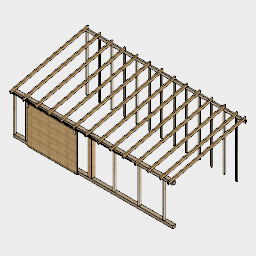
Doro4 Workshop v17 (Autodesk Fusion 360 design; units mm, degrees)
Autodesk Fusion 360 part; units mm, degrees
note: some values were not read from the file. Chosen so that the rebuilt part matches the saved one: which face or edge a step refers to. Set by a fixed rule: which sketch regions a step uses.
sketch "Sketch6" plane through (0, 0, 0) normal (0, 0, 1) x (1, 0, 0)
  line L0 (0, 0) -> (8000, 0)
  line L1 (8000, 0) -> (8000, 120)
  line L2 (8000, 120) -> (0, 120)
  line L3 (0, 120) -> (0, 0)
  dimension "d47" = 8000
  dimension "d51" = 120
  measures "d47" distance of L0.start L0.end
  measures "d51" distance of L0.start L2.end
extrude "Extrude1" add sketch "Sketch6" along normal blind 2200 makes body 1 in component "brick wall"
sketch "Sketch7" plane through (0, 0, 0) normal (1, 0, 0) x (0, 1, 0)
  line L0 (-3775, 0) -> (-3625, 0)
  line L1 (-3625, 0) -> (-3625, -50)
  line L2 (-3625, -50) -> (-3775, -50)
  line L3 (-3775, -50) -> (-3775, 0)
  line L4 (-3700, 0) -> (-3700, -50) construction
  dimension "d52" = 150
  dimension "d53" = 50
  dimension "d56" = 3700
  measures "d52" distance of L0.start L0.end
  measures "d53" distance of L0.start L2.end
  measures "d56" distance of origin L4
extrude "Extrude1'" add sketch "Sketch7" along normal blind 8000 separate body makes body 2 in component "concrete sleepers"
sketch "Sketch8" plane through (0, 0, 0) normal (0, 0, 1) x (1, 0, 0)
  line L0 (-1000, 1000) -> (10000, 1000)
  line L1 (10000, 1000) -> (10000, -7000)
  line L2 (10000, -7000) -> (-1000, -7000)
  line L3 (-1000, -7000) -> (-1000, 1000)
extrude "Extrude1''" add sketch "Sketch8" against normal blind 500 separate body makes body 3 in component "sand"
combine "Combine1" operation cut target body 3 tool bodies 2 keep tools in component "sand"
sketch "Sketch9" plane through (0, 0, 0) normal (1, 0, 0) x (0, 1, 0)
  line L0 (0, 0) -> (-60, 0)
  line L1 (-60, 0) -> (-60, 3000)
  line L2 (-60, 3000) -> (0, 3000)
  line L3 (0, 3000) -> (0, 0)
  line L4 (-3700, 0) -> (-3600, 0)
  line L5 (-3600, 0) -> (-3600, 2150)
  line L6 (-3600, 2150) -> (-3700, 2150)
  line L7 (-3700, 2150) -> (-3700, 0)
  line L8 (-3600, 2150) -> (0, 3000)
  line L9 (-3600, 2150) -> (-3745.9859, 2115.5311)
  line L10 (0, 3000) -> (146.9725, 3034.7018)
  line L11 (120, 0) -> (120, 2200)
  line L12 (-3745.9859, 2115.5311) -> (-3718.4108, 1998.7423)
  line L13 (-3718.4108, 1998.7423) -> (146.9725, 2911.4023)
  line L14 (146.9725, 3034.7018) -> (146.9725, 2911.4023)
  line L15 (146.9725, 3034.7018) -> (141.2276, 3059.0328)
  line L16 (141.2276, 3059.0328) -> (-3849.0547, 2116.8828)
  line L17 (-3849.0547, 2116.8828) -> (-3843.3099, 2092.5518)
  line L18 (-3843.3099, 2092.5518) -> (146.9725, 3034.7018)
  line L19 (-3775, 0) -> (-3625, 0)
  line L20 (0, 2876.7005) -> (-60, 2876.7005)
  line L21 (-60, 2876.7005) -> (-60, 2756.7005)
  line L22 (-60, 2756.7005) -> (0, 2756.7005)
  line L23 (0, 2756.7005) -> (0, 2876.7005)
  line L24 (-3760, 2112.2222) -> (-3600, 2112.2222)
  line L25 (-3600, 2112.2222) -> (-3600, 1952.2222)
  line L26 (-3600, 1952.2222) -> (-3760, 1952.2222)
  line L27 (-3760, 1952.2222) -> (-3760, 2112.2222)
  line L28 (-3575, 2032.6032) -> (-3575, 1952.6032)
  line L29 (-3575, 1952.6032) -> (-3600, 1952.6032)
  point P0 (-3775, 0)
  dimension "d59" = 3000
  dimension "d60" = 60
  dimension "d61" = 2150
  dimension "d62" = 100
  dimension "d63" = 3700
  dimension "d65" = 150
  dimension "d66" = 4000
  dimension "d69" = 13.144
  dimension "d70" = 120
  dimension "d71" = 25
  dimension "d73" = 4100
  dimension "d105" = 60
  dimension "d106" = 120
  dimension "d123" = 160
  dimension "d124" = 160
  dimension "d125" = 80
  dimension "d126" = 25
  measures "d59" distance of L0.start L2.end
  measures "d60" distance of L0.start L0.end
  measures "d61" distance of L4.start L6.end
  measures "d62" distance of L4.start L4.end
  measures "d63" distance of L3 L7
  measures "d65" distance of L5.end L9.end
  measures "d66" distance of L9.end L10.end
  measures "d70" distance of L9.end L12.end
  measures "d71" distance of L10.end L15.end
  measures "d73" distance of L15.end L16.end
  measures "d105" distance of L20.start L20.end
  measures "d106" distance of L20.start L22.end
  measures "d123" distance of L24.start L24.end
  measures "d124" distance of L24.start L26.end
  measures "d125" distance of L28.start L28.end
  measures "d126" distance of L28.end L29.end
extrude "Extrude1'''" add sketch "Sketch9" along normal blind 60 separate body contours L0 L1 L3 L22 | L5 L7 L13 L24 L25 | L5 L7 L13 L25 L26 | L6 L7 L9 L18 | L5 L7 L9 L18 L24 | L4 L5 L7 L19 L26 makes body 4 at (0, -3666.6667, 716.6667) makes body 5 at (40, -60, 918.9002) in component "posts"
copy_body "Body->Comp1" bodies 5 removing the originals makes body 6 in component "KVH 60x60 back"
copy_body "Body->Comp2" bodies 4 removing the originals makes body 7 in component "KVH 100x100 front"
extrude "Extrude1''''" add sketch "Sketch9" along normal blind 60 separate body contours L1 L3 L8 L18 L20 | L3 L10 L13 L14 L18 | L1 L5 L8 L13 L18 L21 L25 | L5 L7 L13 L24 L25 | L5 L7 L9 L18 L24 | L7 L12 L13 L24 | L7 L9 L12 L18 L24 makes body 8 in component "rafter"
extrude "Extrude1'''''" add sketch "Sketch9" along normal blind 8000 separate body contours L1 L2 L8 L18 | L1 L2 L6 L7 L8 L9 L10 L15 L16 L17 L18 | L6 L7 L9 L18 makes body 9 in component "roof deck OSB 25mm"
extrude "Extrude1''''''" add sketch "Sketch9" along normal blind 8000 separate body contours L5 L7 L13 L24 L25 | L5 L7 L13 L25 L26 | L7 L12 L13 L24 | L7 L12 L13 L24 L26 L27 makes body 10 in component "top plate BSH 130x180"
extrude "Extrude1'''''''" add sketch "Sketch9" along normal blind 60 separate body contours L1 L5 L8 L13 L18 L21 L25 makes body 11 in component "knagge OSB 25mm"
extrude "Extrude1''''''''" add sketch "Sketch9" along normal blind 8000 separate body contours L5 L13 L25 L28 L29 makes body 12 in component "sleeper KVH 40x60"
extrude "Extrude1'''''''''" add sketch "Sketch9" along normal blind 8000 separate body contours L1 L3 L13 L21 L22 L23 | L1 L13 L20 L21 makes body 13 in component "top plate KVH 40x60"
sketch "Sketch10" plane through (0, 120, 0) normal (0, 1, 0) x (-1, 0, 0)
  line L0 (-8000, 2100) -> (0, 2100)
  line L1 (0, 2100) -> (0, 3050)
  line L2 (0, 3050) -> (-8000, 3050)
  line L3 (-8000, 3050) -> (-8000, 2100)
  dimension "d107" = 8000
  dimension "d108" = 950
  measures "d107" distance of L0.start L0.end
  measures "d108" distance of L0.start L2.end
extrude "Extrude1''''''''''" add sketch "Sketch10" along normal blind 12 separate body makes body 14 in component "OSB 12mm"
pattern_linear "R-Pattern1" [suppressed] in component "rafters"
sketch "Sketch11" plane through (0, 0, 0) normal (0, 0, -1) x (1, 0, 0)
  line L0 (3750, 3700) -> (3750, 3600)
  line L1 (3750, 3600) -> (3810, 3600)
  line L2 (3810, 3600) -> (3810, 3700)
  line L3 (3810, 3700) -> (3750, 3700)
  line L4 (3750, 3700) -> (3930, 3700)
  line L5 (3930, 3700) -> (3930, 3520)
  line L6 (3930, 3520) -> (3750, 3520)
  line L7 (3750, 3520) -> (3750, 3700)
  dimension "d115" = 180
  dimension "d116" = 180
  measures "d115" distance of L0.start L4.end
  measures "d116" distance of L0.start L6.end
extrude "Extrude1'''''''''''" add sketch "Sketch11" against normal blind 1984.124 separate body makes body 15 in component "post BSH 180x180"
combine "Combine1'" operation cut target body 15 tool bodies 12 10 keep tools in component "post BSH 180x180"
pattern_linear "R-Pattern1'" [suppressed] in component "posts west"
sketch "Sketch12" plane through (0, 0, 0) normal (0, 0, 1) x (1, 0, 0)
move_face "OffsetFaces1" offset -272.7778 1 faces at (20, -3633.3333, 2150) on bodies 7 in component "KVH 100x100 front"
sketch "Sketch13" plane through (0, 0, 0) normal (-1, 0, 0) x (0, -1, 0)
  line L0 (3760, 1952.2222) -> (3760, 2112.2222)
  line L1 (3600, 1952.2222) -> (3760, 1952.2222)
  line L2 (3760, 1952.2222) -> (3790, 1952.2222)
  line L3 (3790, 1952.2222) -> (3790, 1982.2222)
  line L4 (3760, 1982.2222) -> (3760, 1952.2222)
  line L5 (3786, 1956.2222) -> (3764, 1956.2222)
  line L6 (3764, 1956.2222) -> (3764, 1982.2222)
  line L7 (3786, 1982.2222) -> (3786, 1956.2222)
  line L8 (3764, 1982.2222) -> (3760, 1982.2222)
  line L9 (3786.0001, 1982.5) -> (3790.0001, 1982.5)
  line L10 (3790.0001, 1982.5) -> (3790.0001, 2022.5)
  line L11 (3790.0001, 2022.5) -> (3786.0001, 2022.5)
  line L12 (3786.0001, 2022.5) -> (3786.0001, 1982.5)
  line L13 (3795, 1975) -> (3781.0001, 1975)
  line L14 (3781.0001, 1975) -> (3781.0001, 2030.0001)
  line L15 (3781.0001, 2030.0001) -> (3795, 2030.0001)
  line L16 (3795, 2030.0001) -> (3795, 1975)
  line L17 (3795, 1975) -> (3781.0001, 2030.0001) construction
  line L18 (3781.0001, 1975) -> (3795, 2030.0001) construction
  line L19 (3795, 1975) -> (3794.0001, 1975)
  line L20 (3794.0001, 1975) -> (3790.0001, 1982.5)
  line L21 (3781.0001, 1975) -> (3782.0001, 1975)
  line L22 (3786.0001, 1982.5) -> (3782.0001, 1975)
  line L23 (3781.0001, 2002.5) -> (3795, 2002.5)
  line L24 (3786, 1982.2222) -> (3790, 1982.2222)
  line L25 (3795, 1998.5) -> (3781.0001, 1998.5)
  line L26 (3781.0001, 1998.5) -> (3781.0001, 2006.5)
  line L27 (3781.0001, 2006.5) -> (3795, 2006.5)
  line L28 (3795, 2006.5) -> (3795, 1998.5)
  line L29 (3795, 1998.5) -> (3781.0001, 2006.5) construction
  line L30 (3781.0001, 1998.5) -> (3795, 2006.5) construction
  line L31 (3760, 1940) -> (3785, 1940)
  line L32 (3785, 1940) -> (3785, 40)
  line L33 (3785, 40) -> (3760, 40)
  line L34 (3760, 40) -> (3760, 1940)
  line L35 (3760, 1940) -> (3720, 1940)
  line L36 (3720, 1940) -> (3720, 1880)
  line L37 (3720, 1880) -> (3760, 1880)
  line L38 (3760, 1880) -> (3760, 1940)
  line L39 (3760, 40) -> (3720, 40)
  line L40 (3720, 40) -> (3720, 100)
  line L41 (3720, 100) -> (3760, 100)
  line L42 (3760, 100) -> (3760, 40)
  line L43 (3777.0001, 1989.4383) -> (3777.0001, 2032)
  line L44 (3799.0001, 2032) -> (3799.0001, 1732)
  arc A0 (3799.0001, 2032) -> (3777.0001, 2032) centre (3788.0001, 2032) ccw
  line L45 (3775.5001, 1989.4383) -> (3775.5001, 2032)
  arc A1 (3800.5001, 2032) -> (3775.5001, 2032) centre (3788.0001, 2032) ccw
  line L46 (3800.5001, 2032) -> (3800.5001, 1732)
  line L47 (3775.5001, 1989.4383) -> (3777.0001, 1989.4383)
  line L48 (3799.0001, 1732) -> (3800.5001, 1732)
  point P0 (3788.0001, 2002.5)
  point P1 (3788.0001, 2002.5)
  dimension "d128" = 30
  dimension "d129" = 30
  dimension "d132" = 40
  dimension "d134" = 8
  dimension "d135" = 25
  dimension "d136" = 1900
  dimension "d137" = 60
  dimension "d138" = 40
  dimension "d139" = 40
  dimension "d140" = 60
  dimension "d141" = 300
  dimension "d142" = 1.5
  measures "d128" distance of L0.start L2.end
  measures "d129" distance of L0.start L4.start
  measures "d132" distance of L9.start L11.end
  measures "d134" distance of L25.end L26.end
  measures "d135" distance of L31.start L31.end
  measures "d136" distance of L31.start L33.end
  measures "d137" distance of L31.start L37.end
  measures "d138" distance of L31.start L35.end
  measures "d139" distance of L33.end L39.end
  measures "d140" distance of L33.end L41.end
  measures "d141" distance of L44.start L44.end
extrude "Extrude1''''''''''''" add sketch "Sketch13" against normal blind 6000 separate body contours L0 L2 L3 L4 L5 L6 L7 L8 L13 | L3 L7 L13 L24 makes body 16 in component "Component''"
extrude "Extrude1'''''''''''''" add sketch "Sketch13" against normal blind 60 separate body contours L43 L44 A0 L45 A1 L46 L47 L48 makes body 17 in component "Component'''"
revolve "Revolve1" add sketch "Sketch13" angle 360 about axis through (0, -3781.0001, 2002.5) along (0, -1, 0) separate body contours L10 L13 L16 L19 L20 L25 | L9 L10 L12 L25 | L12 L13 L14 L21 L22 L25 makes body 18 in component "Component''''"
extrude "Extrude1''''''''''''''" add sketch "Sketch13" against normal blind 2500 separate body contours L31 L32 L33 L34 L38 L42 makes body 19 in component "Component'''''"
extrude "Extrude1'''''''''''''''" add sketch "Sketch13" against normal blind 2500 separate body contours L34 L35 L36 L37 L38 | L34 L39 L40 L41 L42 makes body 20 at (833.3333, -3760, 1900) makes body 21 at (833.3333, -3760, 60) in component "Component''''''"
move_face "OffsetFaces1'" offset -30 3 faces at (2666.6667, -3666.6667, 2112.2222) (2666.6667, -3730.1365, 2112.2222) (5333.3333, -3755.0682, 2112.2222) on bodies 10 in component "top plate BSH 130x180"
sketch "Sketch14" plane through (7560, 0, 0) normal (1, 0, 0) x (0, 1, 0)
  line L0 (-3700, 0) -> (-3700, 2550)
  line L1 (0, 0) -> (0, 3450)
  line L2 (0, 3450) -> (-3700, 2550)
  line L3 (0, 0) -> (-3700, 0)
  dimension "d153" = 2550
  dimension "d154" = 3450
  measures "d153" distance of L0.start L0.end
  measures "d154" distance of L1.start L1.end
extrude "Extrude1''''''''''''''''" add sketch "Sketch9" along normal blind 8000 separate body contours L5 L7 L13 L24 L25 | L5 L7 L13 L25 L26 | L7 L12 L13 L24 | L7 L12 L13 L24 L26 L27 makes body 22 in component "top plate BSH 130x180 (1)"
move_face "OffsetFaces1''" offset -30 3 faces at (2666.6667, -3666.6667, 2112.2222) (2666.6667, -3730.1365, 2112.2222) (5333.3333, -3755.0682, 2112.2222) on bodies 22 in component "top plate BSH 130x180 (1)"
move_face "OffsetFaces2" offset -130 1 faces at (20, -3666.6667, 0) on bodies 7 in component "KVH 100x100 front"
move_face "OffsetFaces1'''" offset -130 1 faces at (3810, -3640, 0) on bodies 15 in component "post BSH 180x180"
move_face "OffsetFaces1''''" offset -145 1 faces at (20, 146.9725, 2993.602) on bodies 8 in component "rafter"
move_face "OffsetFaces2'" offset 145 2 faces at (20, -3736.2734, 2074.3956) (20, -3745.7255, 2114.4281) on bodies 8 in component "rafter"
extrude "Extrude1'''''''''''''''''" [suppressed] in component "Frame Element"
extrude "Extrude1''''''''''''''''''" [suppressed]
extrude "Extrude2" [suppressed]
sketch "Sketch2" plane through (8100, 0, 0) normal (1, 0, 0) x (0, 1, 0)
  line L0 (-2950, 0) -> (-2950, 2000)
  line L1 (-3450, 0) -> (-3450, 2000)
  line L2 (-2950, 0) -> (-3450, 0)
  line L3 (-2950, 2000) -> (-3450, 2000)
  line L4 (-3450, 0) -> (-3400, 0)
  line L5 (-3400, 0) -> (-3400, 2550)
  line L6 (-3400, 2550) -> (-3450, 2550)
  line L7 (-3450, 2550) -> (-3450, 0)
  line L8 (-100, 0) -> (0, 0)
  line L9 (-100, 0) -> (-100, 2000)
  line L10 (0, 2000) -> (-100, 2000)
  line L11 (0, 0) -> (0, 2000)
  line L12 (-100, 2000) -> (-3450, 2550)
  line L13 (-3450, 2550) -> (-3420.8382, 2727.622)
  line L14 (-100, 2000) -> (-70.8382, 2177.622)
  line L15 (-70.8382, 2177.622) -> (-3420.8382, 2727.622)
  line L16 (-70.8382, 2177.622) -> (-41.2345, 2172.7617)
  line L17 (-41.2345, 2172.7617) -> (0, 2000)
  line L18 (-3420.8382, 2727.622) -> (-3618.196, 2760.0241)
  line L19 (-3450, 2550) -> (-3548.6789, 2566.201)
  line L20 (-3618.196, 2760.0241) -> (-3627.9166, 2700.8167)
  line L21 (-3627.9166, 2700.8167) -> (-3548.6789, 2566.201)
  line L22 (-3450, 0) -> (-3500, 0)
  line L23 (-3500, 0) -> (-3500, 2550)
  line L24 (-3500, 2550) -> (-3450, 2550)
  line L25 (-3450, 2550) -> (-3450, 0)
  dimension "d16" = 2550
  dimension "d17" = 50
  dimension "d18" = 180
  dimension "d19" = 180
  dimension "d20" = 30
  dimension "d21" = 200
  dimension "d22" = 100
  dimension "d23" = 60
  dimension "d26" = 50
  dimension "d46" = 2550
  measures "d16" distance of L1.start L6.end
  measures "d17" distance of L1.start L4.end
  measures "d18" distance of L6.end L13.end
  measures "d19" distance of L9.end L14.end
  measures "d20" distance of L14.end L16.end
  measures "d21" distance of L13.end L18.end
  measures "d22" distance of L6.end L19.end
  measures "d23" distance of L18.end L20.end
  measures "d26" distance of L1.start L22.end
  measures "d46" distance of L22.end L23.end
extrude "Extrude3" [suppressed]
copy_body "CutPasteBodies1" [suppressed] in component "Frame Element"
extrude "Extrude4" [suppressed]
copy_body "CutPasteBodies2" [suppressed] in component "Frame Element"
sketch "Sketch3" plane through (0, 802.823, 1792.9713) normal (0, 0.408665, 0.912685) x (-1, 0, 0)
  line L0 (-8100, 4779.0884) -> (-8040, 4779.0884)
  line L1 (-8100, 4779.0884) -> (-8100, 4679.0884)
  line L2 (-8040, 4679.0884) -> (-8040, 4779.0884)
  line L3 (-8100, 4579.0884) -> (-8100, 4679.0884)
  line L4 (-8040, 4579.0884) -> (-8040, 4679.0884)
  line L5 (-8100, 4533.4541) -> (-8100, 4579.0884)
  line L6 (-8040, 4533.4541) -> (-8040, 4579.0884)
  line L7 (-8100, 4524.3049) -> (-8100, 4533.4541)
  line L8 (-8040, 4524.3049) -> (-8040, 4533.4541)
  line L9 (-8100, 908.5979) -> (-8100, 4524.3049)
  line L10 (-8040, 908.5979) -> (-8040, 4524.3049)
  line L11 (-8100, 817.3295) -> (-8100, 908.5979)
  line L12 (-8040, 817.3295) -> (-8040, 908.5979)
  line L13 (-8100, 817.3295) -> (-8040, 817.3295)
  line L14 (-8100, 4779.0884) -> (400, 4779.0884)
  line L15 (400, 4779.0884) -> (400, 1279.0884)
  line L16 (400, 1279.0884) -> (-8100, 1279.0884)
  line L17 (-8100, 1279.0884) -> (-8100, 4779.0884)
  dimension "d27" = 3500
  dimension "d28" = 8500
  measures "d27" distance of L0.start L16.end
  measures "d28" distance of L0.start L14.end
extrude "Extrude1'''''''''''''''''''" [suppressed] in component "Component"
pattern_linear "R-Pattern1''" [suppressed]
sketch "Sketch4" plane through (-333.3333, 0, 0) normal (-1, 0, 0) x (0, -1, 0)
  line L0 (0, 0) -> (625, 0)
  line L1 (625, 0) -> (625, 2050)
  line L2 (625, 2050) -> (0, 2050)
  line L3 (0, 2050) -> (0, 0)
  dimension "d35" = 625
  dimension "d36" = 2050
  measures "d35" distance of L0.start L0.end
  measures "d36" distance of L0.start L2.end
extrude "Extrude1''''''''''''''''''''" [suppressed] in component "Component'"
sketch "Sketch5" plane through (0, -3500, 0) normal (0, -1, 0) x (1, 0, 0)
  line L0 (8100, 0) -> (5600, 0)
  line L1 (5600, 0) -> (5600, 1250)
  line L2 (5600, 1250) -> (8100, 1250)
  line L3 (8100, 1250) -> (8100, 0)
  dimension "d39" = 2500
  dimension "d40" = 1250
  measures "d39" distance of L0.start L0.end
  measures "d40" distance of L0.start L2.end
extrude "Extrude1'''''''''''''''''''''" [suppressed] in component "OSB 15mm 2500x1250"
extrude "Extrude1''''''''''''''''''''''" [suppressed] in component "OSB 15mm 2500x1250 (1)"
move_face "OffsetFaces1'''''" [suppressed] in component "OSB 15mm 2500x1250 (1)"
extrude "Extrude1'''''''''''''''''''''''" [suppressed] in component "OSB 15mm 2500x1250 (2)"
move_face "OffsetFaces1''''''" [suppressed] in component "OSB 15mm 2500x1250 (2)"
component "brick wall" placed x (1, 0, 0) y (0, 1, 0) z (0, 0, 1) at (0, 0, 0)
component "concrete sleepers" placed x (1, 0, 0) y (0, 1, 0) z (0, 0, 1) at (0, 0, 0)
component "sand" placed x (1, 0, 0) y (0, 1, 0) z (0, 0, 1) at (0, 0, 0)
component "posts" placed x (1, 0, 0) y (0, 1, 0) z (0, 0, 1) at (0, 0, 0)
component "rafter" placed x (1, 0, 0) y (0, 1, 0) z (0, 0, 1) at (0, 0, 0)
component "roof deck OSB 25mm" placed x (1, 0, 0) y (0, 1, 0) z (0, 0, 1) at (0, 0, 0)
component "top plate BSH 130x180" placed x (1, 0, 0) y (0, 1, 0) z (0, 0, 1) at (0, 60, -75)
component "sleeper KVH 40x60" placed x (1, 0, 0) y (0, 1, 0) z (0, 0, 1) at (0, 0, 0)
component "top plate KVH 40x60" placed x (1, 0, 0) y (0, 1, 0) z (0, 0, 1) at (0, 0, 0)
component "OSB 12mm" placed x (1, 0, 0) y (0, 1, 0) z (0, 0, 1) at (0, 0, 0)
component "Rahmen" placed x (1, 0, 0) y (0, 1, 0) z (0, 0, 1) at (5000, 0, 0)
component "Rahmen" placed x (1, 0, 0) y (0, 1, 0) z (0, 0, 1) at (6250, 0, 0)
component "Rahmen" placed x (1, 0, 0) y (0, 1, 0) z (0, 0, 1) at (7500, 0, 0)
component "rafters" placed x (1, 0, 0) y (0, 1, 0) z (0, 0, 1) at (0, 0, 0)
component "post BSH 180x180" placed x (1, 0, 0) y (0, 1, 0) z (0, 0, 1) at (0, 0, 0)
component "post BSH 180x180" placed x (1, 0, 0) y (0, 1, 0) z (0, 0, 1) at (-3125, 0, 0)
component "posts west" placed x (1, 0, 0) y (0, 1, 0) z (0, 0, 1) at (-625, 0, 0)
component "Component''" placed x (1, 0, 0) y (0, 1, 0) z (0, 0, 1) at (0, 0, 0)
component "Component'''" placed x (1, 0, 0) y (0, 1, 0) z (0, 0, 1) at (800, 0, 0)
component "Component''''" placed x (1, 0, 0) y (0, 1, 0) z (0, 0, 1) at (830, 0, 0)
component "Component'''''" placed x (1, 0, 0) y (0, 1, 0) z (0, 0, 1) at (800, -14.0001, 0)
component "Component''''''" placed x (1, 0, 0) y (0, 1, 0) z (0, 0, 1) at (800, -14.0001, 0)
component "Component'''" placed x (1, 0, 0) y (0, 1, 0) z (0, 0, 1) at (3150, 0, 0)
component "Component''''" placed x (1, 0, 0) y (0, 1, 0) z (0, 0, 1) at (3180, 0, 0)
component "top plate BSH 130x180 (1)" placed x (1, 0, 0) y (0, 1, 0) z (0, 0, 1) at (0, 60, -1952.2222)
component "KVH 100x100 front" placed x (1, 0, 0) y (0, 1, 0) z (0, 0, 1) at (0, 0, 0) in component "posts"
component "posts" placed x (1, 0, 0) y (0, 1, 0) z (0, 0, 1) at (0, 0, 0) in component "Rahmen"
component "rafter" placed x (1, 0, 0) y (0, 1, 0) z (0, 0, 1) at (625, 0, 0) in component "rafters"
component "rafter" placed x (1, 0, 0) y (0, 1, 0) z (0, 0, 1) at (1250, 0, 0) in component "rafters"
component "rafter" placed x (1, 0, 0) y (0, 1, 0) z (0, 0, 1) at (1875, 0, 0) in component "rafters"
component "rafter" placed x (1, 0, 0) y (0, 1, 0) z (0, 0, 1) at (2500, 0, 0) in component "rafters"
component "rafter" placed x (1, 0, 0) y (0, 1, 0) z (0, 0, 1) at (3125, 0, 0) in component "rafters"
component "rafter" placed x (1, 0, 0) y (0, 1, 0) z (0, 0, 1) at (3750, 0, 0) in component "rafters"
component "rafter" placed x (1, 0, 0) y (0, 1, 0) z (0, 0, 1) at (4375, 0, 0) in component "rafters"
component "rafter" placed x (1, 0, 0) y (0, 1, 0) z (0, 0, 1) at (5000, 0, 0) in component "rafters"
component "rafter" placed x (1, 0, 0) y (0, 1, 0) z (0, 0, 1) at (5625, 0, 0) in component "rafters"
component "rafter" placed x (1, 0, 0) y (0, 1, 0) z (0, 0, 1) at (6250, 0, 0) in component "rafters"
component "rafter" placed x (1, 0, 0) y (0, 1, 0) z (0, 0, 1) at (6875, 0, 0) in component "rafters"
component "rafter" placed x (1, 0, 0) y (0, 1, 0) z (0, 0, 1) at (7500, 0, 0) in component "rafters"
component "rafter" placed x (1, 0, 0) y (0, 1, 0) z (0, 0, 1) at (7900, 0, 0) in component "rafters"
component "KVH 60x60 back" placed x (1, 0, 0) y (0, 1, 0) z (0, 0, 1) at (625, 0, 0) in component "posts west"
component "KVH 60x60 back" placed x (1, 0, 0) y (0, 1, 0) z (0, 0, 1) at (1250, 0, 0) in component "posts west"
component "KVH 60x60 back" placed x (1, 0, 0) y (0, 1, 0) z (0, 0, 1) at (1875, 0, 0) in component "posts west"
component "KVH 60x60 back" placed x (1, 0, 0) y (0, 1, 0) z (0, 0, 1) at (2500, 0, 0) in component "posts west"
component "KVH 60x60 back" placed x (1, 0, 0) y (0, 1, 0) z (0, 0, 1) at (3125, 0, 0) in component "posts west"
component "KVH 60x60 back" placed x (1, 0, 0) y (0, 1, 0) z (0, 0, 1) at (3750, 0, 0) in component "posts west"
component "KVH 60x60 back" placed x (1, 0, 0) y (0, 1, 0) z (0, 0, 1) at (4375, 0, 0) in component "posts west"
component "KVH 60x60 back" placed x (1, 0, 0) y (0, 1, 0) z (0, 0, 1) at (5000, 0, 0) in component "posts west"
component "KVH 60x60 back" placed x (1, 0, 0) y (0, 1, 0) z (0, 0, 1) at (5625, 0, 0) in component "posts west"
component "KVH 60x60 back" placed x (1, 0, 0) y (0, 1, 0) z (0, 0, 1) at (6250, 0, 0) in component "posts west"
component "KVH 60x60 back" placed x (1, 0, 0) y (0, 1, 0) z (0, 0, 1) at (6875, 0, 0) in component "posts west"
component "KVH 60x60 back" placed x (1, 0, 0) y (0, 1, 0) z (0, 0, 1) at (7500, 0, 0) in component "posts west"
component "KVH 60x60 back" placed x (1, 0, 0) y (0, 1, 0) z (0, 0, 1) at (8125, 0, 0) in component "posts west"
equation "d19 = d18"
equation "d22 = d21 / 2"
equation "d23 = d18 / 3"
equation "d26 = d17"
equation "d33 = ( 2500 / 3 ) * 1 mm"
equation "d43 = ( -2500 / 3 ) * 1 mm"
equation "d44 = ( -2500 / 3 * 2 ) * 1 mm"
equation "d46 = d16"
